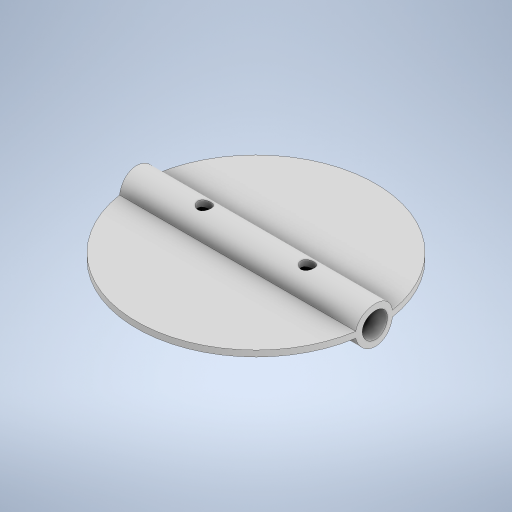
# Autodesk Inventor part: flap
Saved by Autodesk Inventor 2023 (Build 270158000, 158)
## iProperties
Created: 2023-10-25
Part Number: flap
Material: Generic
Document SubType Name: Modeling
Designer: mirek
Density: 1 g/cm^3
Appearance: Default
Author: mirek
Autodesk Inventor part; units mm, degrees
ref_plane "YZ Plane" through (0, 0, 0) normal (1, 0, 0) x (0, 1, 0)
ref_plane "XZ Plane" through (0, 0, 0) normal (0, 1, 0) x (-1, 0, 0)
ref_plane "XY Plane" through (0, 0, 0) normal (0, 0, 1) x (1, 0, 0)
sketch "Sketch1" plane through (0, 0, 0) normal (1, 0, 0) x (0, 1, 0)
  line L0 (-0.25, 9.95) -> (0.25, 9.95)
  line L1 (0.25, -9.95) -> (-0.25, -9.95)
  line L2 (-0.25, 9.95) -> (0.25, -9.95) construction
  line L3 (0.25, 9.95) -> (-0.25, -9.95) construction
  circle A0 centre (0, 0) radius 1.05
  line L4 (0.25, 9.95) -> (0.25, 1.5297)
  line L5 (0.25, -1.5297) -> (0.25, -9.95)
  line L6 (-0.25, -9.95) -> (-0.25, -1.5297)
  line L7 (-0.25, 1.5297) -> (-0.25, 9.95)
  arc A1 (0.25, -1.5297) -> (0.25, 1.5297) centre (0, 0) ccw
  arc A2 (-0.25, 1.5297) -> (-0.25, -1.5297) centre (0, 0) ccw
  dimension "d0" = 0.5
  dimension "d1" = 19.9
  dimension "d3" = 2.1
  dimension "d4" = 0.5
  constraints: 16 end point, 5 parallel, 4 point on circle, 3 centre point, 2 horizontal alignment, 2 midpoint, 2 perpendicular, 1 coincident, 1 horizontal
  measures "d0" distance of L0.start L0.end
  measures "d1" distance of L0.end L1.start
  measures "d3" diameter of A0
  measures "d4" radial gap between concentric circles of A1 A0
extrude "Extrusion1" add sketch "Sketch1" along normal mid plane 19.9
sketch "Sketch2" plane through (0, 0, 0) normal (0, 1, 0) x (-1, 0, 0)
  circle A0 centre (0, 0) radius 9.95
  circle A1 centre (-4.3, 0) radius 0.55
  line L0 (9.95, 1.5297) -> (-9.95, 1.5297) projected
  line L1 (0, 1.5297) -> (0, -1.5297)
  line L2 (-9.95, -1.5297) -> (9.95, -1.5297) projected
  circle A2 centre (4.3, 0) radius 0.55
  dimension "d7" = 19.9
  dimension "d10" = 1.1
  dimension "d11" = 7.5
  constraints: 3 centre point, 2 end point, 2 midpoint, 1 coincident, 1 symmetric about line, 1 other
  measures "d7" diameter of A0
  measures "d10" diameter of A1
extrude "Extrusion2" cut sketch "Sketch2" along normal mid plane 10 keep common part
body "Solid1"
